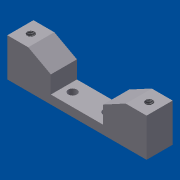
# Autodesk Inventor part: SM-TM1
Saved by Autodesk Inventor 2012 SP1 (Build 160190100, 190)
## iProperties
Created: 2012-04-23
Part Number: SM-TM1
Material: Aluminum-6061
Document SubType Name: Modeling
Designer: ERF
Mass: 37.9787 g
Surface Area: 59.6468 cm^2
Volume: 14.0143 cm^3
Density: 2.71 g/cm^3
Stock Number: SM-TM1
Description: Angled Spindle Mount - piece 1 of 2
Vendor: Shapeoko
Project: Shapeoko
Author: ERF
Title: Spindle Mount
Autodesk Inventor part; units mm, degrees
ref_plane "YZ Plane" through (0, 0, 0) normal (1, 0, 0) x (0, 1, 0)
ref_plane "XZ Plane" through (0, 0, 0) normal (0, 1, 0) x (-1, 0, 0)
ref_plane "XY Plane" through (0, 0, 0) normal (0, 0, 1) x (1, 0, 0)
sketch "Sketch1" plane through (0, 0, 0) normal (0, 0, 1) x (1, 0, 0)
  line L0 (-36.9645, 19.732) -> (-36.9645, -2.268)
  line L1 (-36.9645, -2.268) -> (43.0355, -2.268)
  line L2 (43.0355, -2.268) -> (43.0355, 19.732)
  line L3 (43.0355, 19.732) -> (31.0355, 19.732)
  line L4 (31.0355, 19.732) -> (18.0355, 12.732)
  line L5 (18.0355, 12.732) -> (18.0355, 2.732)
  line L6 (18.0355, 2.732) -> (-11.9645, 2.732)
  line L7 (-11.9645, 2.732) -> (-11.9645, 12.732)
  line L8 (-11.9645, 12.732) -> (-24.9645, 19.732)
  line L9 (-24.9645, 19.732) -> (-36.9645, 19.732)
  dimension "d0" = 22
  dimension "d1" = 80
  dimension "d2" = 90
  dimension "d3" = 12
  dimension "d4" = 90
  dimension "d5" = 12
  dimension "d6" = 25
  dimension "d7" = 55
  dimension "d8" = 22
  dimension "d9" = 15
  dimension "d10" = 15
  dimension "d11" = 5
  constraints: 20 end point, 3 parallel, 2 perpendicular, 1 collinear, 1 vertical
  measures "d0" distance of L0.start L0.end
  measures "d1" distance of L0.end L1.end
  measures "d2" angle of L0 L1
  measures "d3" distance of L2.end L3.end
  measures "d4" angle of L3 L2
  measures "d5" distance of L8.end L0.start
  measures "d6" distance from line of L0 L7.end
  measures "d7" distance from line of L0 L4.end
  measures "d8" distance of L1.end L2.end
  measures "d9" distance from line of L1 L7.end
  measures "d10" distance from line of L1 L4.end
  measures "d11" distance between parallel lines of L1 L6
extrude "Extrusion1" add sketch "Sketch1" along normal blind 15
sketch "Sketch2" plane through (-36.9645, -2.268, 0) normal (0, -1, 0) x (1, 0, 0)
  line L0 (80, 15) -> (0, 15) projected
  line L1 (0, 0) -> (0, 15) projected
  circle A0 centre (30, 7.5) radius 2.5
  circle A1 centre (50, 7.5) radius 2.5
  point P0 (36.9645, 0)
  dimension "d14" = 5
  dimension "d17" = 20
  dimension "d22" = 30
  dimension "d23" = 7.5
  constraints: 2 centre point, 1 horizontal, 2 other
  measures "d14" diameter of A0
  measures "d17" distance of A0.centre A1.centre
  measures "d22" distance from line of L1 A0.centre
  measures "d23" distance from line of L0 A0.centre
extrude "Extrusion2" cut sketch "Sketch2" against normal through all
sketch "Sketch3" plane through (-36.9645, 19.732, 0) normal (0, 1, 0) x (1, 0, 0)
  line L0 (12, 0) -> (0, 0) projected
  line L1 (0, 0) -> (0, -15) projected
  line L2 (68, -15) -> (80, -15) projected
  line L3 (80, 0) -> (80, -15) projected
  line L4 (80, 0) -> (68, 0) projected
  line L5 (68, 0) -> (68, -15) projected
  circle A0 centre (6, -7.5) radius 2.5
  circle A1 centre (74, -7.5) radius 2.5
  point P0 (36.9645, 0)
  dimension "d26" = 5
  dimension "d27" = 7.5
  dimension "d28" = 6
  dimension "d29" = 5
  dimension "d30" = 6
  dimension "d31" = 7.5
  constraints: 2 centre point
  measures "d26" diameter of A0
  measures "d27" distance from line of L0 A0.centre
  measures "d28" distance from line of L1 A0.centre
  measures "d29" diameter of A1
  measures "d30" distance from line of L3 A1.centre
  measures "d31" distance from line of L4 A1.centre
hole "Hole1" at (-30.9645, 19.732, 7.5) at (37.0355, 19.732, 7.5) direction (0, -1, 0) diameter 4.134 end through all thread size "M5x0.8" class "6H" standard "ANSI Metric M Profile"
equation "\"d8\" = d0"
equation "\"d31\" = d27"
body "Solid1"
